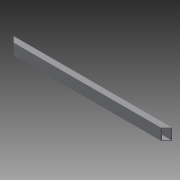
# Autodesk Inventor part: 28in 1x2
Saved by Autodesk Inventor 2015 (Build 190159000, 159)
## iProperties
Created: 2015-01-11
Part Number: 28in 1x2
Material: Generic
Document SubType Name: Modeling
Designer: chapale16
Density: 1 g/cm^3
Appearance: Default
Author: chapale16
Autodesk Inventor part; units mm, degrees
ref_plane "YZ Plane" through (0, 0, 0) normal (1, 0, 0) x (0, 1, 0)
ref_plane "XZ Plane" through (0, 0, 0) normal (0, 1, 0) x (-1, 0, 0)
ref_plane "XY Plane" through (0, 0, 0) normal (0, 0, 1) x (1, 0, 0)
sketch "Sketch1" plane through (0, 0, 0) normal (1, 0, 0) x (0, 1, 0)
  line L0 (10.4423, 8.7344) -> (-40.3577, 8.7344)
  line L1 (-40.3577, 8.7344) -> (-40.3577, -16.6656)
  line L2 (-40.3577, -16.6656) -> (10.4423, -16.6656)
  line L3 (10.4423, -16.6656) -> (10.4423, 8.7344)
  line L4 (7.3181, 5.6102) -> (-37.2335, 5.6102)
  line L5 (-37.2335, 5.6102) -> (-37.2335, -13.5414)
  line L6 (-37.2335, -13.5414) -> (7.3181, -13.5414)
  line L7 (7.3181, -13.5414) -> (7.3181, 5.6102)
  point P0 (0, 0)
  dimension "d0" = 50.8
  dimension "d1" = 25.4
  dimension "d2" = 3.1242
  constraints: 16 end point, 4 parallel, 2 perpendicular, 1 horizontal, 3 other
  measures "d0" distance of L2.end L1.end
  measures "d1" distance of L1.end L0.end
  measures "d2" distance between parallel lines of L3 L7
extrude "Extrusion1" add sketch "Sketch1" along normal blind 711.2
sketch "Sketch2" plane through (0, 10.4423, 8.7344) normal (0, 1, 0) x (1, 0, 0)
  line L0 (0, 25.4) -> (22.2758, 3.1242)
  line L1 (0, 3.1242) -> (711.2, 3.1242) projected
  line L2 (0, 25.4) -> (31.5027, 25.4) construction
  line L3 (22.2758, 3.1242) -> (38.5716, -13.1716)
  line L4 (0, 0) -> (711.2, 0) projected
  line L5 (25.4, 0) -> (0, 0)
  line L6 (0, 0) -> (0, 25.4)
  line L7 (711.2, 25.4) -> (678.2071, -7.5929)
  line L8 (711.2, 25.4) -> (757.859, 25.4) construction
  line L9 (685.8, 0) -> (711.2, 0)
  line L10 (711.2, 0) -> (711.2, 25.4)
  line L11 (711.2, 25.4) -> (711.2, 0) projected
  point P0 (0, 8.7344)
  dimension "d5" = 45
  dimension "d6" = 135
  constraints: 18 end point, 6 point on line, 3 collinear, 2 equal length, 2 horizontal, 1 perpendicular
  measures "d5" angle of L0 L2
  measures "d6" angle of L7 L8
extrude "Extrusion2" cut sketch "Sketch2" against normal blind 711.2 contours L0 L1 L6 | L3 L4 L6 L1
extrude "Extrusion3" cut sketch "Sketch2" against normal blind 711.2 contours L7 L10 L1 | L1 L10 L4 L7
body "Solid1"
